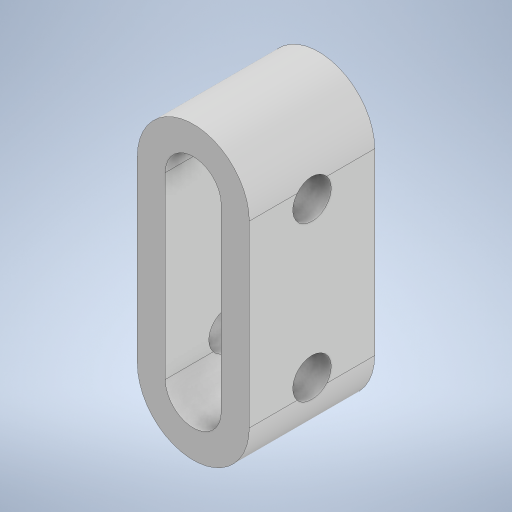
# Autodesk Inventor part: cabeza_obj2
Saved by Autodesk Inventor 2023.2 (Build 272271030, 271C)
## iProperties
Created: 2023-02-25
Part Number: cabeza_obj2
Material: Generic
Document SubType Name: Modeling
Designer: Cris Pat
Density: 1 g/cm^3
Appearance: Default
Author: Cris Pat
Autodesk Inventor part; units mm, degrees
ref_plane "XZ Plane" through (0, 0, 0) normal (0, 1, 0) x (-1, 0, 0)
ref_plane "XY Plane" through (0, 0, 0) normal (0, 0, 1) x (1, 0, 0)
sketch "Sketch1" plane through (0, 0, 0) normal (0, 0, 1) x (1, 0, 0)
  line L0 (-12.5, -20) -> (-12.5, 20)
  arc A0 (12.5, 20) -> (-12.5, 20) centre (0, 20) ccw
  arc A1 (-12.5, -20) -> (12.5, -20) centre (0, -20) ccw
  line L1 (12.5, -20) -> (12.5, 20)
  arc A2 (6.25, 20) -> (-6.25, 20) centre (0, 20) ccw
  arc A3 (-6.25, -20) -> (6.25, -20) centre (0, -20) ccw
  line L2 (6.25, -20) -> (6.25, 20)
  line L3 (-6.25, -20) -> (-6.25, 20)
  point P0 (0, 0)
  point P1 (12.5, 0)
  dimension "d0" = 40
  dimension "d1" = 12.5
  dimension "d2" = 12.5
  constraints: 8 end point, 8 point on circle, 4 centre point, 4 tangent, 3 horizontal alignment, 2 coincident, 2 equal radius, 2 vertical, 1 midpoint, 1 parallel, 1 vertical alignment
  measures "d0" distance of L0.start L0.end
  measures "d1" radius of A0
  measures "d2" diameter of A2
extrude "Extrusion1" add sketch "Sketch1" along normal mid plane 28
ref_plane "Work Plane1" through (12.5, 0, 0) normal (1, 0, 0) x (0, 1, 0)
sketch "Sketch2" plane through (12.5, 0, 0) normal (1, 0, 0) x (0, 1, 0)
  line L0 (20, 14) -> (20, -14) construction
  line L1 (-20, 14) -> (20, 14) construction
  line L2 (-20, -14) -> (-20, 14) construction
  line L3 (20, -14) -> (-20, -14) construction
  circle A0 centre (17.25, 0) radius 4.3
  line L4 (0, 14) -> (0, -14) construction
  line L5 (-20, -14) -> (20, -14) construction
  circle A1 centre (-17.25, 0) radius 4.3
  point P0 (0, 0)
  point P1 (20, 0)
  dimension "d6" = 8.6
  dimension "d7" = 2.75
  constraints: 3 midpoint, 2 centre point, 2 end point, 1 horizontal alignment, 1 symmetric about line, 1 other
  measures "d6" diameter of A0
  measures "d7" distance of A0.centre point (20, 0)
extrude "Extrusion2" cut sketch "Sketch2" against normal blind 28
body "Solid1"
